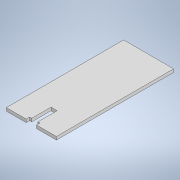
# Autodesk Inventor part: avbay sled
Saved by Autodesk Inventor 2020 (Build 240168000, 168)
## iProperties
Created: 2020-10-12
Part Number: avbay sled
Material: Generic
Document SubType Name: Modeling
Designer: mulve
Density: 1 g/cm^3
Appearance: Default
Author: mulve
Autodesk Inventor part; units mm, degrees
ref_plane "YZ Plane" through (0, 0, 0) normal (1, 0, 0) x (0, 1, 0)
ref_plane "XZ Plane" through (0, 0, 0) normal (0, 1, 0) x (-1, 0, 0)
ref_plane "XY Plane" through (0, 0, 0) normal (0, 0, 1) x (1, 0, 0)
sketch "Sketch1" plane through (0, 0, 0) normal (0, 1, 0) x (-1, 0, 0)
  line L0 (0, 0) -> (48.3455, 0)
  line L1 (48.3455, 0) -> (48.3455, -113.25)
  line L2 (48.3455, -113.25) -> (0, -113.25)
  line L3 (0, -113.25) -> (0, 0)
  line L4 (27.1728, 0) -> (21.1727, 0)
  line L5 (21.1727, 0) -> (21.1727, -21.95)
  line L6 (21.1727, -21.95) -> (27.1728, -21.95)
  line L7 (27.1728, -21.95) -> (27.1728, 0)
  line L8 (29.1728, 0) -> (19.1728, 0)
  line L9 (19.1728, 0) -> (19.1728, -3.302)
  line L10 (19.1728, -3.302) -> (29.1728, -3.302)
  line L11 (29.1728, -3.302) -> (29.1728, 0)
  point P0 (27.1728, -3.302)
  point P1 (21.1727, -3.302)
  dimension "d0" = 113.25
  dimension "d1" = 48.3455
  dimension "d2" = 91.3
  dimension "d3" = 6
  dimension "d4" = 21.1728
  dimension "d5" = 21.1728
  dimension "d6" = 10
  dimension "d7" = 3.302
  dimension "d8" = 2
  dimension "d9" = 2
  constraints: 24 end point, 6 parallel, 3 horizontal, 3 perpendicular, 2 point on line
  measures "d0" distance of L0.end L1.end
  measures "d1" distance of L0.start L0.end
  measures "d2" distance between parallel lines of L2 L6
  measures "d3" distance between parallel lines of L5 L7
  measures "d4" distance between parallel lines of L1 L7
  measures "d5" distance between parallel lines of L3 L5
  measures "d6" distance of L9.end L10.end
  measures "d7" distance between parallel lines of L10 L0
  measures "d8" distance between parallel lines of L5 L9
  measures "d9" distance between parallel lines of L7 L11
extrude "Extrusion1" add sketch "Sketch1" along normal mid plane 3 contours L0 L9 L10 L5 L6 L7 L11 L1 L2 L3
equation "\"d4\" = d5"
equation "\"d8\" = d9"
body "Solid1"
